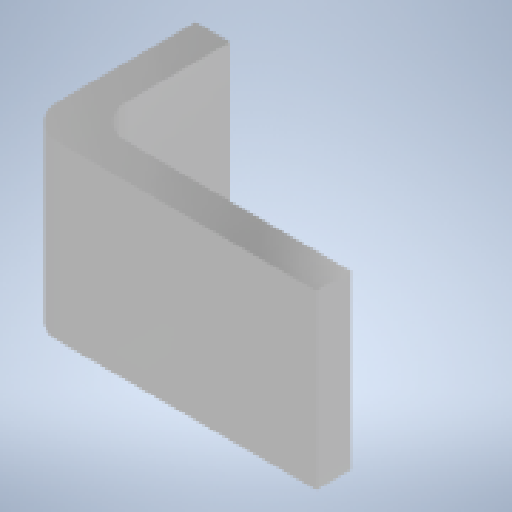
# Autodesk Inventor part: Part4
Saved by Autodesk Inventor 2023 (Build 270158000, 158)
## iProperties
Created: 2023-04-04
Part Number: Part4
Material: Aluminum 6061
Document SubType Name: Modeling
Designer: lukyv
Density: 2.7 g/cm^3
Appearance: Aluminum - Flat
Mass: 17.01 g
Surface Area: 28.285 cm^2
Volume: 6.3 cm^3
Author: lukyv
Autodesk Inventor part; units mm, degrees
ref_plane "YZ Plane" through (0, 0, 0) normal (1, 0, 0) x (0, 1, 0)
ref_plane "XZ Plane" through (0, 0, 0) normal (0, 1, 0) x (-1, 0, 0)
ref_plane "XY Plane" through (0, 0, 0) normal (0, 0, 1) x (1, 0, 0)
sketch "Sketch1" plane through (0, 0, 0) normal (0, 1, 0) x (-1, 0, 0)
  line L0 (-2, 0) -> (-2, 0)
  line L1 (-2, -4) -> (-2, -10)
  line L2 (-2, -10) -> (0, -10)
  line L3 (0, -10) -> (0, -2)
  line L4 (-2, 0) -> (-12, 0)
  line L5 (-12, 0) -> (-12, -2)
  line L6 (-12, -2) -> (-4, -2)
  line L7 (-2, -2) -> (-2, 0)
  arc A0 (-2, -4) -> (-4, -2) centre (-4, -4) ccw
  arc A1 (0, -2) -> (-2, 0) centre (-2, -2) ccw
  point P0 (0, 0)
  dimension "d0" = 2
  dimension "d1" = 2
  dimension "d2" = 10
  dimension "d3" = 10
  dimension "d4" = 2
  dimension "d5" = 2
  constraints: 16 end point, 4 parallel, 4 point on circle, 4 point on line, 4 tangent, 2 centre point, 2 horizontal, 2 perpendicular
  measures "d0" distance of L1.end L2.end
  measures "d1" distance of L4.end L5.end
  measures "d2" distance of L5.end L7.start
  measures "d3" distance of L0.end L1.end
  measures "d4" radius of A0
  measures "d5" radius of A1
extrude "Extrusion1" add sketch "Sketch1" along normal blind 30
equation "\"d1\" = d0"
body "Solid1"
